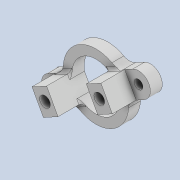
# Autodesk Inventor part: encoder_holder_1
Saved by Autodesk Inventor 2020 (Build 240168000, 168)
## iProperties
Created: 2021-07-15
Part Number: encoder_holder_1
Material: Generic
Document SubType Name: Modeling
Designer: Shuang Peng
Density: 1 g/cm^3
Appearance: Default
Author: Shuang Peng
Autodesk Inventor part; units mm, degrees
ref_plane "YZ Plane" through (0, 0, 0) normal (1, 0, 0) x (0, 1, 0)
ref_plane "XZ Plane" through (0, 0, 0) normal (0, 1, 0) x (-1, 0, 0)
sketch "Sketch1" plane through (0, 0, 0) normal (0, 0, 1) x (1, 0, 0)
  circle A0 centre (0, -4.6) radius 5.15 projected
  line L0 (-7.15, -12.4) -> (-7.15, -10.6) projected
  line L1 (7.15, -12.4) -> (-7.15, -12.4) projected
  line L2 (7.15, -10.6) -> (7.15, -12.4) projected
  line L3 (7.15, -10.6) -> (9.15, -10.6) projected
  line L4 (9.15, -10.6) -> (9.15, 1.4) projected
  line L5 (9.15, 1.4) -> (7.15, 1.4) projected
  line L6 (7.15, 1.4) -> (4.6198, 7.5123) projected
  arc A1 (4.6198, 7.5123) -> (-4.6198, 7.5123) centre (0, 5.6) ccw projected
  line L7 (-4.6198, 7.5123) -> (-7.15, 1.4) projected
  line L8 (-7.15, 1.4) -> (-9.15, 1.4) projected
  line L9 (-9.15, 1.4) -> (-9.15, -10.6) projected
  line L10 (-9.15, -10.6) -> (-7.15, -10.6) projected
  circle A2 centre (7.15, -0.7) radius 0.75 projected
  circle A3 centre (-7.15, -8.5) radius 0.75 projected
  circle A4 centre (-7.15, -0.7) radius 0.75 projected
  circle A5 centre (7.15, -8.5) radius 0.75 projected
  circle A6 centre (0, 5.6) radius 3 projected
  line L11 (-7.15, -8.5) -> (7.15, -0.7) construction
  line L12 (-6.1923, -10.2558) -> (8.1077, -2.4558)
  line L13 (6.1923, 1.0558) -> (-8.1077, -6.7442)
  arc A7 (-8.1077, -6.7442) -> (-6.1923, -10.2558) centre (-7.15, -8.5) ccw
  arc A8 (8.1077, -2.4558) -> (6.1923, 1.0558) centre (7.15, -0.7) ccw
  circle A9 centre (0, -4.6) radius 3.5 projected
  circle A10 centre (0, -4.6) radius 4
  circle A11 centre (0, -4.6) radius 5.5
  point P0 (0, 0)
  point P1 (0, -4.6)
  point P2 (-5.4556, -5.2976)
  point P3 (-3.5402, -8.8092)
  point P4 (5.4556, -3.9024)
  point P5 (3.5402, -0.3908)
  dimension "d0" = 4
  dimension "d1" = 8
  dimension "d2" = 11
  constraints: 8 end point, 4 centre point, 4 point on circle, 4 tangent, 2 coincident, 1 midpoint, 1 parallel
  measures "d0" diameter of A8
  measures "d1" diameter of A10
  measures "d2" diameter of A11
extrude "Extrusion1" add sketch "Sketch1" along normal blind 2 contours A0 L12 A10 | A0 L12 A11 | L12 A10 L13 A0 | A0 L13 A11 L12 | L12 A11 L13 A0 | A0 L13 A10 L12 | L13 A10 A0 | A0 L13 A11 | A11 L13 A8 L12 | L12 A7 L13 A11
sketch "Sketch4" plane through (0, 0, 2) normal (0, 0, 1) x (1, 0, 0)
  arc A0 (3.5402, -0.3908) -> (-5.4556, -5.2976) centre (0, -4.6) ccw projected
  line L0 (-5.4556, -5.2976) -> (-8.1077, -6.7442) projected
  arc A1 (-8.1077, -6.7442) -> (-6.1923, -10.2558) centre (-7.15, -8.5) ccw projected
  line L1 (-6.1923, -10.2558) -> (-3.5402, -8.8092) projected
  arc A2 (-3.5402, -8.8092) -> (5.4556, -3.9024) centre (0, -4.6) ccw projected
  line L2 (5.4556, -3.9024) -> (8.1077, -2.4558) projected
  arc A3 (8.1077, -2.4558) -> (6.1923, 1.0558) centre (7.15, -0.7) ccw projected
  line L3 (6.1923, 1.0558) -> (3.5402, -0.3908) projected
  circle A4 centre (0, -4.6) radius 4 projected
  circle A5 centre (7.15, -0.7) radius 0.75 projected
  circle A6 centre (-7.15, -8.5) radius 0.75 projected
  line L4 (0, -4.6) -> (4.5651, -2.11)
  line L5 (5.4556, -3.9024) -> (8.1077, -2.4558) projected
  line L6 (0, -4.6) -> (-4.5651, -7.09)
  line L7 (-6.1923, -10.2558) -> (-3.5402, -8.8092) projected
  circle A7 centre (4.5651, -2.11) radius 0.9
  circle A8 centre (-4.5651, -7.09) radius 0.9
  point P0 (0, 0)
  dimension "d7" = 5.2
  dimension "d8" = 5.2
  dimension "d9" = 1.8
  dimension "d10" = 1.8
  constraints: 4 end point, 2 centre point, 2 coincident, 2 parallel
  measures "d7" distance of L4.start L4.end
  measures "d8" distance of L4.start L6.end
  measures "d9" diameter of A7
  measures "d10" diameter of A8
extrude "Extrusion3" cut sketch "Sketch4" against normal blind 2 contours A7 | A8
sketch "Sketch5" plane through (0, 0, 2) normal (0, 0, 1) x (1, 0, 0)
  circle A0 centre (-4.5651, -7.09) radius 0.9 projected
  circle A1 centre (4.5651, -2.11) radius 0.9 projected
  arc A2 (3.5402, -0.3908) -> (-5.4556, -5.2976) centre (0, -4.6) ccw projected
  line L0 (-5.4556, -5.2976) -> (-8.1077, -6.7442) projected
  arc A3 (-8.1077, -6.7442) -> (-6.1923, -10.2558) centre (-7.15, -8.5) ccw projected
  line L1 (-6.1923, -10.2558) -> (-3.5402, -8.8092) projected
  arc A4 (-3.5402, -8.8092) -> (5.4556, -3.9024) centre (0, -4.6) ccw projected
  line L2 (5.4556, -3.9024) -> (8.1077, -2.4558) projected
  arc A5 (8.1077, -2.4558) -> (6.1923, 1.0558) centre (7.15, -0.7) ccw projected
  line L3 (6.1923, 1.0558) -> (3.5402, -0.3908) projected
  circle A6 centre (0, -4.6) radius 4 projected
  circle A7 centre (7.15, -0.7) radius 0.75 projected
  circle A8 centre (-7.15, -8.5) radius 0.75 projected
  line L4 (4.8364, 0.3162) -> (6.7518, -3.1954)
  line L5 (6.7518, -3.1954) -> (4.2937, -4.5362)
  line L6 (4.2937, -4.5362) -> (2.3783, -1.0246)
  line L7 (2.3783, -1.0246) -> (4.8364, 0.3162)
  line L8 (4.8364, 0.3162) -> (4.2937, -4.5362) construction
  line L9 (6.7518, -3.1954) -> (2.3783, -1.0246) construction
  line L10 (5.4556, -3.9024) -> (8.1077, -2.4558) projected
  line L11 (-4.2937, -4.6638) -> (-2.3783, -8.1754)
  line L12 (-2.3783, -8.1754) -> (-4.8364, -9.5162)
  line L13 (-4.8364, -9.5162) -> (-6.7518, -6.0046)
  line L14 (-6.7518, -6.0046) -> (-4.2937, -4.6638)
  line L15 (-4.2937, -4.6638) -> (-4.8364, -9.5162) construction
  line L16 (-2.3783, -8.1754) -> (-6.7518, -6.0046) construction
  line L17 (-6.1923, -10.2558) -> (-3.5402, -8.8092) projected
  point P0 (0, 0)
  point P1 (-2.7379, -7.5161)
  point P2 (-3.9341, -5.3231)
  point P3 (2.7379, -1.6839)
  point P4 (3.9341, -3.8769)
  point P5 (5.4556, -3.9024)
  point P6 (6.7518, -3.1954)
  dimension "d13" = 4
  dimension "d14" = 2.8
  dimension "d15" = 4
  dimension "d16" = 2.8
  constraints: 24 end point, 4 midpoint, 4 parallel, 3 perpendicular, 1 collinear
  measures "d13" distance of L4.start L4.end
  measures "d14" distance of L4.end L5.end
  measures "d15" distance of L11.start L11.end
  measures "d16" distance of L11.end L12.end
extrude "Extrusion4" add sketch "Sketch5" against normal blind 2 contours A6 L6 | L11 A6
ref_plane "Work Plane1" through (-7.1257, -10.1802, 4.25) normal (0, 0, -1) x (-0.4788521, 0.8778956, 0)
extrude "Extrusion5" add sketch "Sketch5" along normal blind 4 contours L3 L4 L2 L5 L6 A6 L7 | L14 L11 A6 L12 L1 L13 L0 | A6 L6 | L11 A6
fillet "Fillet1" radius 2 4 edges at (-5.4556, -5.2976, 1) (3.5402, -0.3908, 1) (-3.5402, -8.8092, 1) (5.4556, -3.9024, 1)
fillet "Fillet2" radius 0.5 12 edges at (5.9915, -3.6101, 2) (4.8746, -4.2193, 2) (4.1139, -4.2065, 2) (4.076, -0.0985, 2) (2.9592, -0.7077, 2) (2.5581, -1.3542, 2) (-5.9915, -5.5899, 2) (-4.8746, -4.9807, 2) (-4.1139, -4.9935, 2) (-4.076, -9.1015, 2) (-2.9592, -8.4923, 2) (-2.5581, -7.8458, 2)
body "Solid1"
